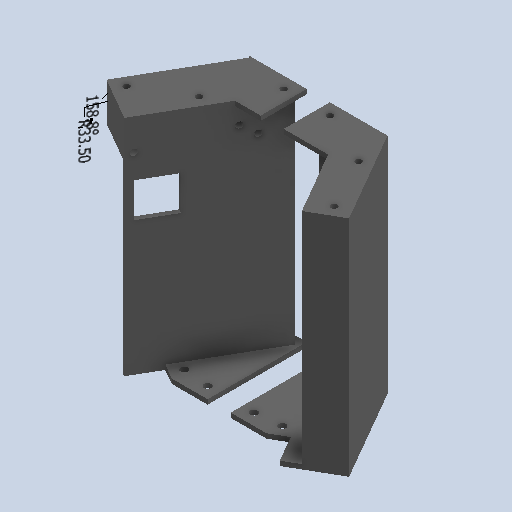
# Autodesk Inventor part: flame_back
Saved by Autodesk Inventor 2024.1 (Build 281209000, 209)
## iProperties
Created: 2025-03-04
Part Number: flame_back
Material: 一般
Document SubType Name: Modeling
Designer: hibik
Density: 1 g/cm^3
Appearance: 既定
Author: hibik
Autodesk Inventor part; units mm, degrees
ref_plane "YZ Plane" through (0, 0, 0) normal (1, 0, 0) x (0, 1, 0)
ref_plane "XZ Plane" through (0, 0, 0) normal (0, 1, 0) x (-1, 0, 0)
ref_plane "XY Plane" through (0, 0, 0) normal (0, 0, 1) x (1, 0, 0)
sketch "スケッチ1" plane through (0, 0, 0) normal (0, 1, 0) x (-1, 0, 0)
  line L0 (-52.75, 39.4042) -> (-30, 0)
  line L1 (-30, 0) -> (0, 0)
  line L2 (-52.75, 39.4042) -> (-39.7596, 46.9042)
  line L3 (-39.7596, 46.9042) -> (-12.6795, 0)
  line L4 (0, -23.8693) -> (0, 62.7831) projected
  line L5 (52.75, 39.4042) -> (30, 0)
  line L6 (30, 0) -> (0, 0)
  line L7 (52.75, 39.4042) -> (39.7596, 46.9042)
  line L8 (39.7596, 46.9042) -> (12.6795, 0)
  line L9 (52.75, 39.4042) -> (35.4295, 49.4042)
  line L10 (35.4295, 49.4042) -> (12.9295, 10.433)
  line L11 (12.9295, 10.433) -> (30.25, 0.433)
  line L12 (30.25, 0.433) -> (52.75, 39.4042)
  line L13 (39.7596, 46.9042) -> (33.6974, 50.4042)
  line L14 (33.6974, 50.4042) -> (0, -7.9615)
  line L15 (12.6795, 0) -> (0, 7.3205)
  point P0 (6.6173, 3.5)
  point P1 (4.5966, 0)
  dimension "d0" = 45.5
  dimension "d1" = 30
  dimension "d2" = 60
  dimension "d3" = 15
  dimension "d40" = 20
  dimension "d41" = 45
  dimension "d65" = 2
  constraints: 30 end point, 6 parallel, 4 symmetric about line, 3 perpendicular, 3 point on line, 2 collinear, 1 coincident, 1 horizontal
  measures "d0" distance from line of L0.end L2
  measures "d1" distance of L0.end L1.end
  measures "d2" angle of L1 L0
  measures "d3" distance between parallel lines of L0 L3
  measures "d40" distance between parallel lines of L10 L12
  measures "d41" distance between parallel lines of L9 L11
  measures "d65" distance between parallel lines of L14 L10
extrude "押し出し1" add sketch "スケッチ1" along normal blind 97 contours L2 L3 L1 L0 | L8 L11 L5 L6 | L15 L14 L13 L10 L11 L8
ref_plane "作業平面1" through (0, 2, 0) normal (0, -1, 0) x (1, 0, 0)
sketch "スケッチ2" plane through (0, 2, 0) normal (0, -1, 0) x (1, 0, 0)
  line L0 (52.75, 39.4042) -> (30, 0) projected
  line L1 (39.7596, 46.9042) -> (52.75, 39.4042) projected
  line L2 (12.6795, 0) -> (39.7596, 46.9042) projected
  line L3 (30, 0) -> (12.6795, 0) projected
  line L4 (-35.4295, 49.4042) -> (-33.6974, 50.4042) projected
  line L5 (-30, 0) -> (-30.25, 0.433) projected
  line L6 (-12.6795, 0) -> (-30, 0) projected
  line L7 (39.0096, 45.6051) -> (49.4019, 39.6051)
  line L8 (49.4019, 39.6051) -> (28.2679, 3)
  line L9 (28.2679, 3) -> (-28.2679, 3)
  line L10 (-28.2679, 3) -> (-49.4019, 39.6051)
  line L11 (-49.4019, 39.6051) -> (-39.0096, 45.6051)
  line L12 (0, -23.8693) -> (0, 62.7831) projected
  line L13 (-33.6974, 50.4042) -> (-6.6173, 3.5) projected
  line L14 (-12.9295, 10.433) -> (-35.4295, 49.4042) projected
  line L15 (-30.25, 0.433) -> (-12.9295, 10.433) projected
  line L16 (-6.6173, 3.5) -> (-12.6795, 0) projected
  point P0 (0, 0)
  point P1 (14.4115, 3)
  dimension "d7" = 1.5
  dimension "d8" = 3
  dimension "d9" = 3
  constraints: 10 end point, 5 parallel, 1 horizontal, 1 perpendicular, 1 point on line, 2 other
  measures "d7" distance between parallel lines of L4 L11
  measures "d8" distance between parallel lines of L6 L9
  measures "d9" distance between parallel lines of L5 L10
extrude "押し出し2" cut sketch "スケッチ2" against normal blind 75 contours L7 L8 L9 L2
sketch "スケッチ4" plane through (49.4019, 2, 39.6051) normal (-0.8660254, 0, 0.5) x (0.5, 0, 0.8660254)
  line L0 (-42.2679, 0) -> (0, 0) projected
  line L1 (0, 0) -> (0, 75) projected
  line L2 (0, 75) -> (-42.2679, 75) projected
  line L3 (-42.2679, 0) -> (-42.2679, 75) projected
  line L4 (-21.134, 75) -> (-21.134, 0) construction
  line L5 (0, 37.5) -> (-42.2679, 37.5) construction
  circle A0 centre (-40, 70) radius 1.35
  circle A1 centre (-5, 70) radius 1.35
  circle A2 centre (-5, 5) radius 1.35
  circle A3 centre (-40, 5) radius 1.35
  point P0 (-59, -2)
  dimension "d14" = 2.7
  dimension "d15" = 2.7
  dimension "d16" = 2.7
  dimension "d17" = 2.7
  dimension "d18" = 35
  dimension "d19" = 65
  dimension "d20" = 5
  constraints: 4 centre point, 4 end point, 4 midpoint, 2 horizontal alignment, 2 symmetric about line, 1 vertical alignment
  measures "d14" diameter of A0
  measures "d15" diameter of A1
  measures "d16" diameter of A2
  measures "d17" diameter of A3
  measures "d18" distance of A1.centre A0.centre
  measures "d19" distance of A2.centre A1.centre
  measures "d20" distance from line of L1 A1.centre
ref_plane "作業平面2" through (45.0718, 2, 42.1051) normal (-0.8660254, 0, 0.5) x (0.5, 0, 0.8660254)
sketch "スケッチ5" plane through (45.0718, 2, 42.1051) normal (-0.8660254, 0, 0.5) x (0.5, 0, 0.8660254)
  circle A0 centre (-40, 70) radius 1.35 projected
  circle A1 centre (-5, 70) radius 1.35 projected
  circle A2 centre (-5, 5) radius 1.35 projected
  circle A3 centre (-40, 5) radius 1.35 projected
  line L0 (-49.1962, 75) -> (0, 75) projected
  line L1 (-49.1962, 0) -> (-49.1962, 75) projected
  line L2 (-42.2679, 0) -> (-42.2679, 75) projected
  line L3 (-36, 75) -> (-46, 75)
  line L4 (-46, 75) -> (-46, 66)
  line L5 (-46, 66) -> (-36, 66)
  line L6 (-36, 66) -> (-36, 75)
  line L7 (-9, 75) -> (1.5, 75)
  line L8 (1.5, 75) -> (1.5, 66)
  line L9 (1.5, 66) -> (-9, 66)
  line L10 (-9, 66) -> (-9, 75)
  line L11 (-9, 0) -> (1.5, 0)
  line L12 (1.5, 0) -> (1.5, 9)
  line L13 (1.5, 9) -> (-9, 9)
  line L14 (-9, 9) -> (-9, 0)
  line L15 (-36, 0) -> (-46, 0)
  line L16 (-46, 0) -> (-46, 9)
  line L17 (-46, 9) -> (-36, 9)
  line L18 (-36, 9) -> (-36, 0)
  line L19 (-42.2679, 0) -> (0, 0) projected
  circle A4 centre (-40, 5) radius 4
  circle A5 centre (-5, 5) radius 4
  line L20 (1.5, -2) -> (1.5, 95) projected
  circle A6 centre (-40, 70) radius 4
  circle A7 centre (-5, 70) radius 4
  point P0 (-59, -2)
  point P1 (-40, 9)
  point P2 (-36, 5)
  point P3 (-5, 9)
  point P4 (-9, 5)
  point P5 (-5, 66)
  point P6 (-9, 70)
  point P7 (-40, 66)
  point P8 (-36, 70)
  dimension "d22" = 8
  dimension "d24" = 10
  constraints: 32 end point, 8 parallel, 7 tangent, 6 point on line, 4 centre point, 4 coincident, 4 horizontal, 4 perpendicular, 3 equal radius, 2 collinear
  measures "d22" diameter of A4
  measures "d24" distance of L15.start L15.end
extrude "押し出し3" add sketch "スケッチ5" against normal up to surface (8 mm away) contours L0 L7 L8 L9 A7 L10 | A7 | L12 L11 L14 A5 L13 | A5
extrude "押し出し4" add sketch "スケッチ5" against normal blind 10 contours L0 L2 A6 L5 L4 | L0 L6 A6 L2 | A6 L2 | L2 A6 | L2 A6 L5 | L17 A4 L2 | L2 A4 L15 L16 L17 | A4 L2 | L2 A4 | A4 L18 L15 L2
sketch "スケッチ8" plane through (0, 97, 0) normal (0, 1, 0) x (1, 0, 0)
  line L0 (34, -6.9282) -> (30, 0) projected
  line L1 (34, -6.9282) -> (35.7321, -5.9282) projected
  line L2 (30.7321, 2.7321) -> (35.7321, -5.9282) projected
  line L3 (26, 0) -> (30.7321, 2.7321) projected
  line L4 (30, 0) -> (26, 0) projected
  point P0 (0, 0)
extrude "押し出し7" cut sketch "スケッチ8" against normal through all
sketch "スケッチ15" plane through (0, 97, 0) normal (0, 1, 0) x (1, 0, 0)
  line L0 (-12.9295, -10.433) -> (-35.4295, -49.4042) projected
  line L1 (-35.4295, -49.4042) -> (-33.6974, -50.4042) projected
  line L2 (-33.6974, -50.4042) -> (-6.6173, -3.5) projected
  line L3 (-12.6795, 0) -> (-30, 0) projected
  line L4 (-30, 0) -> (-30.25, -0.433) projected
  line L5 (-30.25, -0.433) -> (-12.9295, -10.433) projected
  line L6 (-30.25, -0.433) -> (-52.75, -39.4042)
  line L7 (-52.75, -39.4042) -> (-35.4295, -49.4042)
  line L8 (-6.6173, -3.5) -> (-12.6795, 0) projected
  point P0 (0, 0)
  constraints: 4 end point, 2 perpendicular
extrude "押し出し13" add sketch "スケッチ15" against normal blind 7
sketch "スケッチ16" plane through (-30, 0, 0) normal (-0.8660254, 0, -0.5) x (-0.5, 0, 0.8660254)
  line L0 (0, 0) -> (0, 97) projected
  line L1 (0, 0) -> (0.5, 0) projected
  line L2 (0.5, 0) -> (0.5, 90) projected
  line L3 (45.5, 90) -> (0.5, 90) projected
  line L4 (45.5, 97) -> (45.5, 90) projected
  line L5 (0, 97) -> (45.5, 97) projected
  line L6 (0.5, 90) -> (0, 90)
  point P0 (-15, 0)
  constraints: 2 end point, 1 perpendicular, 1 point on line
extrude "押し出し14" cut sketch "スケッチ16" against normal blind 1 contours L0 L5 L4 L3 L6
sketch "スケッチ18" plane through (-30, 0, 0) normal (-0.8660254, 0, -0.5) x (-0.5, 0, 0.8660254)
  line L0 (0.5, 0) -> (45.5, 0) projected
  line L1 (0.5, 30) -> (0.5, 60) projected
  line L2 (0.5, 65) -> (0, 65) projected
  line L3 (0, 60) -> (0.5, 60) projected
  line L4 (0, 30) -> (0.5, 30) projected
  line L5 (0.5, 25) -> (0, 25) projected
  line L6 (0.5, 0) -> (0.5, 25) projected
  line L7 (0.5, 0) -> (0.5, 90) projected
  line L8 (0.5, 65.5) -> (-2.5, 65.5)
  line L9 (-2.5, 65.5) -> (-2.5, 59.5)
  line L10 (-2.5, 59.5) -> (0.5, 59.5)
  line L11 (0.5, 59.5) -> (0.5, 65.5)
  line L12 (-5, 68) -> (-2, 68)
  line L13 (-2, 68) -> (-2, 57)
  line L14 (-2, 57) -> (-5, 57)
  line L15 (-5, 57) -> (-5, 68)
  line L16 (0.5, 30.5) -> (-2.5, 30.5)
  line L17 (-2.5, 30.5) -> (-2.5, 24.5)
  line L18 (-2.5, 24.5) -> (0.5, 24.5)
  line L19 (0.5, 24.5) -> (0.5, 30.5)
  line L20 (-5, 33) -> (-2, 33)
  line L21 (-2, 33) -> (-2, 22)
  line L22 (-2, 22) -> (-5, 22)
  line L23 (-5, 22) -> (-5, 33)
  line L24 (0, 30) -> (0, 25) projected
  line L25 (0, 65) -> (0, 60) projected
  line L26 (0.5, 65) -> (0.5, 80) projected
  line L27 (45.5, 80) -> (45.5, 0) projected
  line L28 (-2.5, 60) -> (-2.5, 57.5) projected
  line L29 (-2.5, 57.5) -> (-4.5, 57.5) projected
  line L30 (-4.5, 57.5) -> (-4.5, 67.5) projected
  line L31 (-4.5, 67.5) -> (-2.5, 67.5) projected
  line L32 (-2.5, 67.5) -> (-2.5, 65) projected
  line L33 (-2.5, 65) -> (0, 65) projected
  line L34 (0, 25) -> (-2.5, 25) projected
  line L35 (-2.5, 25) -> (-2.5, 22.5) projected
  line L36 (-2.5, 22.5) -> (-4.5, 22.5) projected
  line L37 (-4.5, 22.5) -> (-4.5, 32.5) projected
  line L38 (-4.5, 32.5) -> (-2.5, 32.5) projected
  line L39 (-2.5, 32.5) -> (-2.5, 30) projected
  line L40 (-2.5, 30) -> (0, 30) projected
  line L41 (25.7358, 80) -> (0.5, 80) projected
  line L42 (35.8747, 80) -> (35.8747, 75) projected
  line L43 (35.8747, 75) -> (25.7358, 75) projected
  line L44 (25.7358, 75) -> (25.7358, 80) projected
  line L45 (45.5, 80) -> (35.8747, 80) projected
  point P0 (-15, 0)
  point P1 (-3.5, 33)
  point P2 (-5, 27.5)
  point P3 (-5, 62.5)
  point P4 (-3.5, 68)
  point P5 (-2, 30.5)
  point P6 (-2, 24.5)
  point P7 (0.5, 24.5)
  point P8 (0.5, 65.2)
  point P9 (-2, 65.5)
  point P10 (-2, 59.5)
  point P11 (0.5, 60)
  point P12 (0.5, 60)
  point P13 (45.5, 84.6044)
  point P14 (0.5, 84.6044)
  point P15 (-3.5, 67.5)
  point P16 (-4.5, 62.5)
  point P17 (-4.5, 27.5)
  point P18 (-3.5, 32.5)
  dimension "d99" = 0.5
  dimension "d100" = 0.5
  dimension "d101" = 0.5
  dimension "d102" = 0.5
  dimension "d149" = 0.5
  dimension "d150" = 0.5
  dimension "d151" = 0.5
  dimension "d152" = 0.5
  constraints: 32 end point, 8 midpoint, 8 parallel, 4 horizontal, 4 perpendicular, 2 collinear, 2 horizontal alignment, 2 point on line, 2 vertical alignment
  measures "d99" distance between parallel lines of L16 L4
  measures "d100" distance between parallel lines of L18 L5
  measures "d101" distance between parallel lines of L8 L2
  measures "d102" distance between parallel lines of L10 L3
  measures "d149" distance between parallel lines of L12 L31
  measures "d150" distance between parallel lines of L15 L30
  measures "d151" distance between parallel lines of L20 L38
  measures "d152" distance between parallel lines of L23 L37
extrude "押し出し16" cut sketch "スケッチ18" against normal up to surface (20 mm away) contours L18 L21 L34 L5 L6 | L5 L24 L4 L7 | L21 L22 L23 L20 L16 L39 L38 L37 L36 L35 L18 | L18 L17 L34 L21 | L34 L21 L40 L24 | L4 L40 L21 L16 L1 | L35 L36 L37 L38 L39 L17 | L34 L17 L40 L21 | L40 L17 L16 L21 | L10 L13 L33 L25 L3 L1 | L3 L25 L2 L7 | L13 L14 L15 L12 L8 L32 L31 L30 L29 L28 L10 | L10 L9 L33 L13 | L2 L33 L13 L8 L7 | L28 L29 L30 L31 L32 L9 | L33 L9 L8 L13
sketch "スケッチ19" plane through (0, 97, 0) normal (0, 1, 0) x (1, 0, 0)
  line L0 (-30, 0) -> (30, 0) projected
  line L1 (-58.25, -48.9304) -> (-30, 0) projected
  line L2 (-30, -65.2406) -> (-58.25, -48.9304) projected
  line L3 (-30, -20) -> (-30, -65.2406) projected
  line L4 (30, -20) -> (-30, -20) projected
  line L5 (30, -65.2406) -> (30, -20) projected
  line L6 (58.25, -48.9304) -> (30, -65.2406) projected
  line L7 (30, 0) -> (58.25, -48.9304) projected
  line L8 (5, -20) -> (-5, -20)
  line L9 (-5, -20) -> (-5, 0)
  line L10 (-5, 0) -> (5, 0)
  line L11 (5, 0) -> (5, -20)
  line L12 (12.6795, 0) -> (39.7596, -46.9042) projected
  line L13 (-33.6974, -50.4042) -> (-6.6173, -3.5) projected
  line L14 (-6.6173, -3.5) -> (-12.6795, 0) projected
  line L15 (0, -20) -> (0, 0)
  line L16 (33.6974, -50.4042) -> (6.6173, -3.5)
  line L17 (6.6173, -3.5) -> (12.6795, 0)
  line L18 (14.4115, -3) -> (22.4944, -3) projected
  line L19 (14.4115, -3) -> (39.0096, -45.6051) projected
  line L20 (14.4115, -3) -> (8.3494, -6.5)
  circle A0 centre (34.5994, -57.9663) radius 1.6 projected
  circle A1 centre (-34.5994, -57.9663) radius 1.6 projected
  circle A2 centre (-47.5897, -50.4663) radius 1.6 projected
  circle A3 centre (47.5897, -50.4663) radius 1.6 projected
  circle A4 centre (0, -16) radius 1.6 projected
  circle A5 centre (0, -4) radius 1.6 projected
  circle A6 centre (10, -15.9234) radius 1.6 projected
  circle A7 centre (-10, -15.9234) radius 1.6 projected
  circle A8 centre (-10, -5) radius 1.6 projected
  circle A9 centre (10, -5) radius 1.6 projected
  circle A10 centre (45.0538, -38.074) radius 1.6 projected
  circle A11 centre (33.4199, -15.9234) radius 1.6 projected
  circle A12 centre (-45.0538, -38.074) radius 1.6 projected
  point P0 (0, 0)
  point P1 (0, 0)
  point P2 (-16.1436, -20)
  point P3 (24.2265, -20)
  dimension "d105" = 10
  constraints: 16 end point, 5 point on line, 3 midpoint, 3 perpendicular, 2 parallel, 2 symmetric about line, 1 coincident, 1 horizontal
  measures "d105" distance between parallel lines of L9 L11
extrude "押し出し17" add sketch "スケッチ19" against normal blind 2 contours L0 L9 L4 L13 L14 | L0 L17 L16 L4 L11 | L12 L20 A9 L16 L17 | L12 L4 L16 L20 A9 | A9 L20 | L20 A9 | A6 | A7
sketch "スケッチ20" plane through (0, 97, 0) normal (0, 1, 0) x (1, 0, 0)
  line L0 (-6.6173, -3.5) -> (-16.1436, -20) projected
  line L1 (-12.6795, 0) -> (-5, 0) projected
  line L2 (-12.6795, 0) -> (-6.6173, -3.5) projected
  line L3 (0, 0) -> (0, -11.75)
  line L4 (6.6173, -3.5) -> (16.1436, -20)
  line L5 (12.6795, 0) -> (6.6173, -3.5)
  line L6 (14.4115, -3) -> (22.4944, -3) projected
  line L7 (12.6795, 0) -> (14.4115, -3)
  line L8 (24.2265, -20) -> (12.6795, 0) projected
  line L9 (14.4115, -3) -> (8.3494, -6.5)
  constraints: 10 end point, 3 symmetric about line, 1 collinear, 1 perpendicular, 1 point on line, 1 vertical
extrude "押し出し18" add sketch "スケッチ20" against normal up to surface (97 mm away)
sketch "スケッチ21" plane through (0, 0, 0) normal (0, -1, 0) x (1, 0, 0)
  line L0 (-33.6974, 50.4042) -> (-6.6173, 3.5)
  line L1 (0, 0) -> (0, 12.9111)
  line L2 (33.6974, 50.4042) -> (6.6173, 3.5)
  line L3 (33.6974, 50.4042) -> (39.7596, 46.9042)
  line L4 (39.0096, 45.6051) -> (14.4115, 3)
  line L5 (14.4115, 3) -> (39.7596, 46.9042)
  line L6 (25.3673, 45.976) -> (-25.3673, 45.976)
  line L7 (27.1974, 39.1458) -> (20.5635, 42.976)
  line L8 (20.5635, 42.976) -> (-20.5635, 42.976)
  line L9 (-20.5635, 42.976) -> (-27.1974, 39.1458)
  line L10 (5, 20) -> (5, 0)
  line L11 (-5, 0) -> (-5, 20)
  line L12 (5, 20) -> (24.2265, 20)
  line L13 (5, 20) -> (5, 42.976)
  line L14 (-5, 20) -> (-5, 42.976)
  line L15 (6.6173, 3.5) -> (12.6795, 0)
  line L16 (-6.6173, 3.5) -> (-12.6795, 0)
  line L17 (52.75, 39.4042) -> (30, 0)
  line L18 (39.7596, 46.9042) -> (52.75, 39.4042)
  line L19 (14.4115, 3) -> (39.7596, 46.9042)
  line L20 (14.4115, 3) -> (8.3494, 6.5)
  line L21 (8.3494, 6.5) -> (6.6173, 3.5)
  line L22 (6.6173, 3.5) -> (12.6795, 0)
  line L23 (30, 0) -> (12.6795, 0)
  line L24 (30, 0) -> (-30, 0)
  line L25 (-30, 0) -> (-48.75, 32.476)
  line L26 (-30.25, 0.433) -> (-52.75, 39.4042)
  line L27 (-52.75, 39.4042) -> (-35.4295, 49.4042)
  line L28 (-12.9295, 10.433) -> (-35.4295, 49.4042)
  line L29 (-30.25, 0.433) -> (-12.9295, 10.433)
  line L30 (-30, 0) -> (-30.25, 0.433)
  line L31 (-12.6795, 0) -> (-30, 0)
  line L32 (-6.6173, 3.5) -> (-12.6795, 0)
  line L33 (-33.6974, 50.4042) -> (-6.6173, 3.5)
  line L34 (-35.4295, 49.4042) -> (-33.6974, 50.4042)
extrude "押し出し19" add sketch "スケッチ21" against normal blind 2 contours L0 L16 L24 L25 L29 L28 L34 | L9 L8 L14 L11 L24 L16 L0 | L8 L7 L2 L12 L13 | L12 L2 L15 L24 L10 | L2 L3 L5 L4 L12 | L12 L4 L20 L2 | L15 L2 L20 L4 L5 L18 L17 L23
sketch "スケッチ22" plane through (0, 0, 0) normal (0, -1, 0) x (1, 0, 0)
  circle A0 centre (-10, 37.976) radius 1.6
  circle A1 centre (-21.2333, 36.8157) radius 1.6
  circle A2 centre (-10, 5) radius 1.35
  line L0 (-5, 0) -> (-5, 42.976) projected
  line L1 (-20.5635, 42.976) -> (-27.1974, 39.1458) projected
  line L2 (-5, 42.976) -> (-20.5635, 42.976) projected
  line L3 (-12.9295, 10.433) -> (-35.4295, 49.4042) projected
  line L4 (-30, 0) -> (-5, 0) projected
  point P0 (0, 0)
  dimension "d114" = 3.2
  dimension "d115" = 5
  dimension "d116" = 5
  dimension "d117" = 5
  dimension "d118" = 6
  dimension "d119" = 5
  dimension "d125" = 2.7
  constraints: 3 centre point, 1 equal radius, 1 vertical alignment
  measures "d114" diameter of A0
  measures "d115" distance from line of L0 A0.centre
  measures "d116" distance from line of L1 A1.centre
  measures "d117" distance from line of L2 A0.centre
  measures "d118" distance from line of L3 A1.centre
  measures "d119" distance from line of L4 A2.centre
  measures "d125" diameter of A2
extrude "押し出し20" cut sketch "スケッチ22" against normal up to surface (2 mm away)
sketch "スケッチ23" plane through (0, 0, 0) normal (0, -1, 0) x (1, 0, 0)
  circle A0 centre (-10, 5) radius 1.35 projected
  circle A1 centre (-10, 5) radius 1.35
  point P0 (0, 0)
  dimension "d122" = 2.7
  constraints: 1 centre point, 1 coincident
  measures "d122" diameter of A1
extrude "押し出し21" cut sketch "スケッチ23" against normal blind 10
sketch "スケッチ25" plane through (0, 97, 0) normal (0, 1, 0) x (1, 0, 0)
  circle A0 centre (-25.5276, -26.2535) radius 1.35
  circle A1 centre (-10, -5) radius 1.35
  circle A2 centre (-45.0538, -38.074) radius 1.35
  line L0 (-51.884, -39.9042) -> (-33.6974, -50.4042) projected
  line L1 (-29.134, -0.5) -> (-51.884, -39.9042) projected
  line L2 (-35.4295, -49.4042) -> (-12.9295, -10.433) projected
  line L3 (-33.6974, -50.4042) -> (-16.1436, -20) projected
  line L4 (-5, -20) -> (-5, 0) projected
  line L5 (-5, 0) -> (-30, 0) projected
  point P0 (0, 0)
  point P1 (-47.259, -31.8934)
  dimension "d126" = 2.7
  dimension "d127" = 5
  dimension "d128" = 5
  dimension "d129" = 5
  dimension "d130" = 25
  dimension "d131" = 5
  dimension "d132" = 5
  constraints: 3 centre point, 2 equal radius
  measures "d126" diameter of A2
  measures "d127" distance from line of L0 A2.centre
  measures "d128" distance from line of L1 A2.centre
  measures "d129" distance from line of L3 A0.centre
  measures "d130" distance from line of L0 A0.centre
  measures "d131" distance from line of L4 A1.centre
  measures "d132" distance from line of L5 A1.centre
extrude "押し出し22" cut sketch "スケッチ25" against normal blind 10
mirror "ミラー2" about plane through (0, 0, 0) normal (1, 0, 0) of "押し出し20", "押し出し21", "押し出し22"
sketch "スケッチ26" plane through (0, 2, 0) normal (0, 1, 0) x (1, 0, 0)
  line L0 (11.3317, -4.7782) -> (14.4115, -3) projected
  line L1 (11.3317, -4.7782) -> (14.4115, -3) projected
  line L2 (11.3317, -4.7782) -> (9.1421, -6.0423) projected
  line L3 (8.3494, -6.5) -> (9.1421, -6.0423) projected
  line L4 (8.3494, -6.5) -> (9.1421, -6.0423) projected
  line L5 (9.1421, -6.0423) -> (11.3317, -4.7782) projected
  arc A0 (9.1421, -6.0423) -> (11.3317, -4.7782) centre (10, -5) ccw projected
  line L6 (8.3494, -6.5) -> (14.4115, -3)
  line L7 (14.4115, -3) -> (16.4115, -6.4641)
  line L8 (16.4115, -6.4641) -> (10.3494, -9.9641)
  line L9 (10.3494, -9.9641) -> (8.3494, -6.5)
  line L10 (11.3317, -4.7782) -> (14.4115, -3) projected
  point P0 (0, 0)
  point P1 (14.4115, -3)
  point P2 (12.8716, -3.8891)
  dimension "d135" = 4
  constraints: 8 end point, 2 parallel, 1 midpoint, 1 perpendicular
  measures "d135" distance from line of point (12.872, -3.889) L8
extrude "押し出し23" add sketch "スケッチ26" along normal blind 15 contours L0 L7 L8 L9 L3 A0
sketch "スケッチ27" plane through (0, 95, 0) normal (0, -1, 0) x (1, 0, 0)
  line L0 (10.3494, 9.9641) -> (16.4115, 6.4641) projected
  line L1 (16.4115, 6.4641) -> (14.4115, 3) projected
  line L2 (11.3317, 4.7782) -> (14.4115, 3) projected
  arc A0 (11.3317, 4.7782) -> (9.1421, 6.0423) centre (10, 5) ccw projected
  line L3 (8.3494, 6.5) -> (9.1421, 6.0423) projected
  line L4 (8.3494, 6.5) -> (10.3494, 9.9641) projected
  point P0 (0, 0)
extrude "押し出し24" add sketch "スケッチ27" along normal up to surface (18 mm away)
sketch "スケッチ28" plane through (0, 97, 0) normal (0, 1, 0) x (1, 0, 0)
  circle A0 centre (33.4199, -15.9234) radius 1.35
  circle A1 centre (10, -5) radius 1.35 projected
  line L0 (24.2265, -20) -> (39.7596, -46.9042) projected
  line L1 (52.75, -39.4042) -> (30, 0) projected
  line L2 (39.7596, -46.9042) -> (52.75, -39.4042) projected
  point P0 (0, 0)
  dimension "d141" = 5
  dimension "d142" = 30
  constraints: 1 centre point, 1 equal radius
  measures "d141" distance from line of L1 A0.centre
  measures "d142" distance from line of L2 A0.centre
extrude "押し出し25" cut sketch "スケッチ28" against normal blind 10 contours A0
sketch "スケッチ30" plane through (-33.6974, 0, 50.4042) normal (0.8660254, 0, 0.5) x (0.5, 0, -0.8660254)
  line L0 (3, 58) -> (18, 58) projected
  line L1 (18, 58) -> (18, 78) projected
  line L2 (3, 0) -> (42, 0) projected
  line L3 (3, 0) -> (3, 58) projected
  line L4 (18, 58) -> (3, 58)
  line L5 (3, 58) -> (3, 73)
  line L6 (3, 73) -> (18, 73)
  line L7 (18, 73) -> (18, 58)
  point P0 (60.5, 0)
  point P1 (18, 73)
  point P2 (3, 58)
  dimension "d189" = 15
  constraints: 8 end point, 2 collinear, 2 parallel, 1 horizontal, 1 perpendicular, 1 point on line
  measures "d189" distance of L4.end L5.end
extrude "押し出し27" cut sketch "スケッチ30" against normal up to surface (2 mm away)
ref_plane "作業平面3" through (0, 80.5, 0) normal (0, -1, 0) x (1, 0, 0)
sketch "スケッチ31" plane through (0, 90, 0) normal (0, -1, 0) x (1, 0, 0)
  circle A0 centre (-45.0538, 38.074) radius 1.35 projected
  circle A1 centre (-25.5276, 26.2535) radius 1.35 projected
  line L0 (-51.884, 39.9042) -> (-29.384, 0.933) projected
  line L1 (-12.9295, 10.433) -> (-29.384, 0.933) projected
  line L2 (-35.4295, 49.4042) -> (-12.9295, 10.433) projected
  line L3 (-35.4295, 49.4042) -> (-51.884, 39.9042) projected
  point P0 (0, 0)
extrude "押し出し28" add sketch "スケッチ31" along normal up to surface (9.5 mm away)
sketch "スケッチ32" plane through (-29.134, 0, 0.5) normal (-0.8660254, 0, -0.5) x (-0.5, 0, 0.8660254)
  circle A0 centre (5, 93.5) radius 2.5
  line L0 (5, 93.5) -> (38.5, 80.5)
  line L1 (0.5, 80.5) -> (45.5, 80.5) projected
  line L2 (38.5, 93.5) -> (38.5, 80.5)
  line L3 (41.85, 97) -> (41.85, 80.5) projected
  line L4 (38.5, 93.5) -> (5, 93.5)
  line L5 (0, 97) -> (45.5, 97) projected
  line L6 (45.5, 97) -> (45.5, 80.5) projected
  line L7 (0, 90) -> (0, 97) projected
  line L8 (5, 95.5) -> (38.5, 95.5)
  line L9 (38.5, 95.5) -> (38.5, 93.5)
  line L10 (0.5186, 94.1664) -> (35.7358, 80.5)
  arc A1 (35.8552, 80.4537) -> (38.5, 93.5) centre (5, 93.5) ccw
  line L11 (25.7358, 84.3806) -> (25.7358, 80.5)
  point P0 (-15, 0)
  point P1 (6.5, 95.5)
  point P2 (6.7743, 91.7388)
  point P3 (35.8747, 80.5)
  point P4 (36.2309, 81.3805)
  dimension "d158" = 5
  dimension "d159" = 3.5
  dimension "d160" = 7
  dimension "d161" = 5
  dimension "d162" = 2
  dimension "d163" = 1
  dimension "d166" = 10
  constraints: 14 end point, 5 point on line, 2 centre point, 2 horizontal, 2 parallel, 2 perpendicular, 2 point on circle, 1 coincident, 1 tangent
  measures "d158" diameter of A0
  measures "d159" distance from line of L5 L0.start
  measures "d160" distance between parallel lines of L6 L2
  measures "d161" distance from line of L7 L0.start
  measures "d162" distance between parallel lines of L8 L4
  measures "d163" distance between parallel lines of L10 L0
  measures "d166" distance from line of L10.end L11
extrude "押し出し29" cut sketch "スケッチ32" against normal blind 5 contours L4 L0 A0 L10 | L4 A1 L0 A0 | A0 L8 L9 L4 | A0 L0 L4 | L0 A1 L1 L10 A0 | L10 A0 | L10 L1 L11
sketch "スケッチ33" plane through (-24.8038, 0, 3) normal (-0.8660254, 0, -0.5) x (-0.5, 0, 0.8660254)
  line L0 (25.7358, 84.3806) -> (6.7743, 91.7388) projected
  line L1 (25.7358, 80.5) -> (25.7358, 84.3806) projected
  line L2 (35.8747, 80.5) -> (25.7358, 80.5) projected
  arc A0 (35.8747, 80.5) -> (38.5, 93.5) centre (5, 93.5) ccw projected
  line L3 (38.5, 95.5) -> (38.5, 93.5) projected
  line L4 (6.5, 95.5) -> (38.5, 95.5) projected
  arc A1 (6.5, 95.5) -> (6.7743, 91.7388) centre (5, 93.5) ccw projected
  circle A2 centre (5, 93.5) radius 2.5
  arc A3 (6.5, 95.5) -> (6.7743, 91.7388) centre (5, 93.5) ccw projected
  point P0 (-15, 0)
  point P1 (6.7743, 91.7388)
  point P2 (6.5, 95.5)
  constraints: 1 centre point, 1 coincident, 1 concentric
extrude "押し出し30" cut sketch "スケッチ33" against normal blind 5 contours A1 A2
sketch "スケッチ34" plane through (-29.134, 0, 0.5) normal (-0.8660254, 0, -0.5) x (-0.5, 0, 0.8660254)
  arc A0 (35.8747, 80.5) -> (38.5, 93.5) centre (5, 93.5) ccw projected
  line L0 (35.8747, 80.5) -> (45.5, 80.5) projected
  line L1 (45.5, 97) -> (45.5, 80.5) projected
  line L2 (0, 97) -> (45.5, 97) projected
  line L3 (0, 90) -> (0, 97) projected
  line L4 (0.5, 90) -> (0, 90) projected
  line L5 (0.5, 80.5) -> (0.5, 90) projected
  line L6 (0.5, 80.5) -> (25.7358, 80.5) projected
  line L7 (25.7358, 80.5) -> (25.7358, 84.3806) projected
  line L8 (25.7358, 84.3806) -> (6.7743, 91.7388) projected
  arc A1 (6.5, 95.5) -> (6.7743, 91.7388) centre (5, 93.5) ccw projected
  line L9 (6.5, 95.5) -> (38.5, 95.5) projected
  line L10 (38.5, 95.5) -> (38.5, 93.5) projected
  line L11 (0.5, 90) -> (0, 90)
  line L12 (0, 90) -> (0, 80.5)
  line L13 (0, 80.5) -> (0.5, 80.5)
  line L14 (0.5, 80.5) -> (0.5, 90)
  line L15 (0.5, 80.5) -> (25.7358, 80.5) projected
  line L16 (0, 90) -> (0, 97) projected
  point P0 (-15, 0)
  point P1 (0.5, 80.5)
  point P2 (0, 90)
  constraints: 8 end point, 2 collinear, 2 parallel, 1 horizontal, 1 perpendicular
extrude "押し出し31" cut sketch "スケッチ34" along normal up to surface (1 mm away) contours L4 L5 L13 L12
sketch "スケッチ35" plane through (-29.134, 0, 0.5) normal (-0.8660254, 0, -0.5) x (-0.5, 0, 0.8660254)
  circle A0 centre (3, 83.5) radius 1.35
  circle A1 centre (42.5, 83.5) radius 1.35
  circle A2 centre (9, 87.6571) radius 1.35
  line L0 (25.7358, 84.3806) -> (6.7743, 91.7388) projected
  line L1 (45.5, 97) -> (45.5, 80.5) projected
  line L2 (35.8747, 80.5) -> (45.5, 80.5) projected
  line L3 (0.5, 80.5) -> (25.7358, 80.5) projected
  line L4 (0, 80.5) -> (0, 97) projected
  arc A3 (6.5, 95.5) -> (6.7743, 91.7388) centre (5, 93.5) ccw projected
  point P0 (-15, 0)
  dimension "d176" = 2.7
  dimension "d177" = 3
  dimension "d178" = 3
  dimension "d179" = 3
  dimension "d180" = 3
  dimension "d181" = 3
  dimension "d182" = 4
  constraints: 3 centre point, 2 equal radius
  measures "d176" diameter of A0
  measures "d177" distance from line of L0 A2.centre
  measures "d178" distance from line of L1 A1.centre
  measures "d179" distance from line of L2 A1.centre
  measures "d180" distance from line of L3 A0.centre
  measures "d181" distance from line of L4 A0.centre
  measures "d182" horizontal distance of A3.centre A2.centre
extrude "押し出し32" cut sketch "スケッチ35" against normal up to surface (21 mm away)
sketch "スケッチ36" plane through (-12.9295, 30.5, 10.433) normal (-0.5, 0, 0.8660254) x (0.8660254, 0, 0.5)
  line L0 (-20, 22) -> (-14, 22)
  line L1 (-14, 22) -> (-14, 7)
  line L2 (-14, 7) -> (-20, 7)
  line L3 (-20, 7) -> (-20, 22)
  line L4 (-20, 0) -> (-20, 29) projected
  line L5 (-20, 0) -> (-20, 29) projected
  point P0 (5.9808, -30.5)
  point P1 (-20, 14.5)
  point P2 (-20, 14.5)
  dimension "d185" = 15
  dimension "d186" = 6
  constraints: 8 end point, 2 midpoint, 2 parallel, 1 coincident, 1 collinear, 1 horizontal, 1 perpendicular
  measures "d185" distance of L2.end L0.start
  measures "d186" distance of L0.start L0.end
extrude "押し出し33" cut sketch "スケッチ36" against normal through all
equation "\"d99\" = d151"
equation "\"d100\" = d99"
equation "\"d101\" = d149"
equation "\"d102\" = d101"
equation "\"d149\" = d150"
equation "\"d151\" = d150"
equation "\"d152\" = d151"
equation "\"d117\" = d115"
equation "\"d119\" = d117"
